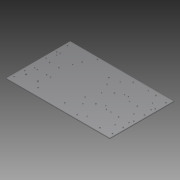
# Autodesk Inventor part: Rebuild Mounting Board 1
Saved by Autodesk Inventor 2014 SP1 (Build 180222100, 222)
## iProperties
Created: 2013-01-21
Part Number: Rebuild Mounting Board 1
Material: Polycarbonate, Clear
Document SubType Name: Modeling
Designer: Moses
Density: 1.2 g/cm^3
Mass: 569.716 g
Surface Area: 3066.4 cm^2
Volume: 474.763 cm^3
Appearance: Polycarbonate - Clear
Author: Moses
Autodesk Inventor part; units mm, degrees
ref_plane "YZ Plane" through (0, 0, 0) normal (1, 0, 0) x (0, 1, 0)
ref_plane "XZ Plane" through (0, 0, 0) normal (0, 1, 0) x (-1, 0, 0)
ref_plane "XY Plane" through (0, 0, 0) normal (0, 0, 1) x (1, 0, 0)
sketch "Sketch1" plane through (0, 0, 0) normal (0, 1, 0) x (-1, 0, 0)
  line L0 (0, 0) -> (493.7125, 0)
  line L1 (493.7125, 0) -> (493.7125, 304.8)
  line L2 (0, 304.8) -> (0, 0)
  line L3 (0, 304.8) -> (493.7125, 304.8)
  circle A0 centre (42.8625, 236.5375) radius 1.905
  circle A1 centre (104.9909, 194.7291) radius 1.905
  line L4 (38.1, 241.3) -> (109.7534, 241.3) construction
  line L5 (109.7534, 241.3) -> (109.7534, 189.9666) construction
  line L6 (109.7534, 189.9666) -> (38.1, 189.9666) construction
  line L7 (38.1, 189.9666) -> (38.1, 241.3) construction
  circle A2 centre (252.4125, 266.7) radius 2.54
  circle A3 centre (379.4125, 266.7) radius 2.54
  circle A4 centre (252.4125, 57.15) radius 2.54
  circle A5 centre (379.4125, 57.15) radius 2.54
  line L8 (252.4125, 266.7) -> (379.4125, 266.7) construction
  line L9 (379.4125, 266.7) -> (379.4125, 57.15) construction
  line L10 (379.4125, 57.15) -> (252.4125, 57.15) construction
  line L11 (252.4125, 266.7) -> (252.4125, 57.15) construction
  line L12 (481.0125, 304.8) -> (481.0125, 0) construction
  circle A6 centre (481.0125, 279.4) radius 2.54
  line L13 (12.7, 304.8) -> (12.7, 0) construction
  circle A7 centre (12.7, 279.4) radius 2.54
  circle A8 centre (481.0125, 228.6) radius 2.54
  circle A9 centre (12.7, 228.6) radius 2.54
  circle A10 centre (481.0125, 177.8) radius 2.54
  circle A11 centre (12.7, 177.8) radius 2.54
  circle A12 centre (481.0125, 127) radius 2.54
  circle A13 centre (12.7, 127) radius 2.54
  circle A14 centre (66.675, 285.4833) radius 2.54
  line L14 (406.0013, 241.3) -> (461.9625, 241.3) construction
  circle A15 centre (406.0013, 241.3) radius 3.302
  circle A16 centre (461.9625, 241.3) radius 3.302
  circle A17 centre (455.6125, 136.017) radius 2.54
  circle A18 centre (455.6125, 194.183) radius 2.54
  circle A19 centre (411.1625, 136.017) radius 2.54
  circle A20 centre (411.1625, 194.183) radius 2.54
  line L15 (455.6125, 136.017) -> (455.6125, 194.183) construction
  line L16 (411.1625, 136.017) -> (411.1625, 194.183) construction
  line L17 (411.1625, 165.1) -> (455.6125, 165.1) construction
  circle A21 centre (468.3125, 9.525) radius 2.54
  circle A22 centre (481.0125, 76.2) radius 2.54
  circle A23 centre (12.7, 76.2) radius 2.54
  circle A24 centre (481.0125, 25.4) radius 2.54
  circle A25 centre (12.7, 25.4) radius 2.54
  circle A26 centre (468.3125, 73.025) radius 2.54
  circle A27 centre (354.0125, 9.525) radius 2.54
  circle A28 centre (354.0125, 73.025) radius 2.54
  circle A29 centre (206.5909, 226.4791) radius 1.905
  circle A30 centre (144.4625, 268.2875) radius 1.905
  line L18 (139.7, 273.05) -> (211.3534, 273.05) construction
  line L19 (211.3534, 273.05) -> (211.3534, 221.7166) construction
  line L20 (211.3534, 221.7166) -> (139.7, 221.7166) construction
  line L21 (139.7, 221.7166) -> (139.7, 273.05) construction
  circle A31 centre (174.625, 285.4833) radius 2.54
  circle A32 centre (66.675, 196.5833) radius 2.54
  circle A33 centre (174.625, 196.5833) radius 2.54
  circle A34 centre (66.675, 107.6833) radius 2.54
  circle A35 centre (174.625, 107.6833) radius 2.54
  circle A36 centre (66.675, 18.7833) radius 2.54
  circle A37 centre (174.625, 18.7833) radius 2.54
  line L22 (144.4625, 268.2875) -> (206.5909, 268.2875) construction
  line L23 (206.5909, 268.2875) -> (206.5909, 226.4791) construction
  line L24 (206.5909, 226.4791) -> (144.4625, 226.4791) construction
  line L25 (144.4625, 226.4791) -> (144.4625, 268.2875) construction
  line L26 (42.8625, 236.5375) -> (104.9909, 236.5375) construction
  line L27 (104.9909, 236.5375) -> (104.9909, 194.7291) construction
  line L28 (104.9909, 194.7291) -> (42.8625, 194.7291) construction
  line L29 (42.8625, 194.7291) -> (42.8625, 236.5375) construction
  circle A38 centre (42.8625, 147.6375) radius 1.905
  circle A39 centre (104.9909, 105.8291) radius 1.905
  line L30 (38.1, 152.4) -> (109.7534, 152.4) construction
  line L31 (109.7534, 152.4) -> (109.7534, 101.0666) construction
  line L32 (109.7534, 101.0666) -> (38.1, 101.0666) construction
  line L33 (38.1, 101.0666) -> (38.1, 152.4) construction
  circle A40 centre (42.8625, 58.7375) radius 1.905
  circle A41 centre (104.9909, 16.9291) radius 1.905
  line L34 (38.1, 63.5) -> (109.7534, 63.5) construction
  line L35 (109.7534, 63.5) -> (109.7534, 12.1666) construction
  line L36 (109.7534, 12.1666) -> (38.1, 12.1666) construction
  line L37 (38.1, 12.1666) -> (38.1, 63.5) construction
  circle A42 centre (206.5909, 137.5791) radius 1.905
  circle A43 centre (144.4625, 179.3875) radius 1.905
  line L38 (139.7, 184.15) -> (211.3534, 184.15) construction
  line L39 (211.3534, 184.15) -> (211.3534, 132.8166) construction
  line L40 (211.3534, 132.8166) -> (139.7, 132.8166) construction
  line L41 (139.7, 132.8166) -> (139.7, 184.15) construction
  circle A44 centre (206.5909, 48.6791) radius 1.905
  circle A45 centre (144.4625, 90.4875) radius 1.905
  line L42 (139.7, 95.25) -> (211.3534, 95.25) construction
  line L43 (211.3534, 95.25) -> (211.3534, 43.9166) construction
  line L44 (211.3534, 43.9166) -> (139.7, 43.9166) construction
  line L45 (139.7, 43.9166) -> (139.7, 95.25) construction
  circle A46 centre (19.05, 194.183) radius 2.2479 projected
  circle A47 centre (127, 194.183) radius 2.2479 projected
  circle A48 centre (228.6, 194.183) radius 2.2479 projected
  circle A49 centre (392.1252, 194.183) radius 2.2479 projected
  circle A50 centre (468.3252, 194.183) radius 2.2479 projected
  circle A51 centre (468.3252, 89.2969) radius 2.2479 projected
  circle A52 centre (392.1252, 89.2969) radius 2.2479 projected
  circle A53 centre (228.6, 89.2969) radius 2.2479 projected
  circle A54 centre (127, 89.2969) radius 2.2479 projected
  circle A55 centre (19.05, 89.2969) radius 2.2479 projected
  dimension "d0" = 304.8
  dimension "d4" = 493.7125
  dimension "d11" = 4.7625
  dimension "d12" = 4.7625
  dimension "d13" = 4.7625
  dimension "d14" = 4.7625
  dimension "d15" = 63.5
  dimension "d17" = 209.55
  dimension "d18" = 127
  dimension "d20" = 114.3
  dimension "d21" = 57.15
  dimension "d32" = 12.7
  dimension "d33" = 5.08
  dimension "d34" = 25.4
  dimension "d35" = 12.7
  dimension "d37" = 25.4
  dimension "d43" = 50.8
  dimension "d57" = 55.9612
  dimension "d59" = 241.3
  dimension "d67" = 165.1
  dimension "d68" = 31.75
  dimension "d69" = 58.166
  dimension "d70" = 44.45
  dimension "d71" = 25.4
  dimension "d81" = 5.08
  dimension "d85" = 9.525
  dimension "d88" = 63.5
  dimension "d91" = 114.3
  dimension "d94" = 25.4
  dimension "d96" = 4.7625
  dimension "d97" = 4.7625
  dimension "d98" = 4.7625
  dimension "d99" = 4.7625
  dimension "d100" = 31.75
  dimension "d103" = 19.3167
  dimension "d104" = 66.675
  dimension "d107" = 107.95
  dimension "d110" = 88.9
  dimension "d113" = 41.8084
  dimension "d114" = 62.1284
  dimension "d115" = 3.81
  dimension "d116" = 101.6
  dimension "d117" = 5.08
  dimension "d118" = 6.604
  dimension "d119" = 5.08
  dimension "d120" = 38.1
  dimension "d121" = 5.08
  dimension "d124" = 88.9
  dimension "d131" = 88.9
  constraints: 92 end point, 46 centre point, 15 parallel, 11 equal radius, 9 horizontal, 8 perpendicular, 7 vertical, 6 point on line, 2 coincident, 2 midpoint, 1 collinear, 87 other
  measures "d0" distance of L2.start L0.start
  measures "d4" distance of L0.start L0.end
  measures "d11" distance from line of L4 L26.start
  measures "d12" distance from line of L26.start L7
  measures "d13" distance from line of L6 L27.end
  measures "d14" distance from line of L5 L27.end
  measures "d15" distance between parallel lines of L3 L4
  measures "d17" distance of L10.end L8.start
  measures "d18" distance of L8.start L8.end
  measures "d20" distance between parallel lines of L1 L9
  measures "d21" distance between parallel lines of L0 L10
  measures "d32" distance between parallel lines of L1 L12
  measures "d33" diameter of A6
  measures "d34" distance from line of A6.centre L3
  measures "d35" distance between parallel lines of L13 L2
  measures "d37" distance from line of L3 A7.centre
  measures "d43" distance of A7.centre A9.centre
  measures "d57" distance of L14.start L14.end
  measures "d59" distance between parallel lines of L0 L14
  measures "d67" distance between parallel lines of L0 L17
  measures "d68" distance from line of L1 L14.end
  measures "d69" distance of L16.start L16.end
  measures "d70" distance of L17.start L17.end
  measures "d71" distance between parallel lines of L12 L15
  measures "d81" diameter of A21
  measures "d85" distance from line of L0 A21.centre
  measures "d88" distance of A21.centre A26.centre
  measures "d91" distance of A21.centre A27.centre
  measures "d94" distance from line of L1 A21.centre
  measures "d96" distance from line of L19 L23.end
  measures "d97" distance from line of L20 L23.end
  measures "d98" distance from line of L18 L22.start
  measures "d99" distance from line of L21 L22.start
  measures "d100" distance between parallel lines of L3 L18
  measures "d103" distance from line of L3 A14.centre
  measures "d104" distance from line of L2 A14.centre
  measures "d107" distance of A14.centre A31.centre
  measures "d110" distance of A14.centre A32.centre
  measures "d113" distance of L26.end L27.end
  measures "d114" distance of L27.end L28.end
  measures "d115" diameter of A0
  measures "d116" distance between parallel lines of L19 L5
  measures "d117" diameter of A2
  measures "d118" diameter of A15
  measures "d119" diameter of A17
  measures "d120" distance between parallel lines of L2 L7
  measures "d121" diameter of A14
  measures "d124" distance of L26.start A38.centre
  measures "d131" distance of L22.start A43.centre
extrude "Extrusion1" add sketch "Sketch1" along normal blind 3.175 contours L2 L3 L1 L0 | A10 | A21 | A28
equation "\"d11\" = d12"
equation "\"d13\" = d12"
equation "\"d14\" = d12"
equation "\"d37\" = d34"
body "Solid1"
